Autodesk Fusion 360 part; units mm, degrees
note: some values were not read from the file. Set by a fixed rule: which sketch regions a step uses.
(part 2 of 4)
  line L656 (1.808, 3.3438) -> (1.8184, 3.3438)
  line L657 (1.8184, 3.3438) -> (1.8184, 3.2708)
  line L658 (1.8184, 3.2708) -> (1.9955, 3.2708)
  line L659 (1.1056, 1.5849) -> (1.0838, 1.7478)
  line L660 (0.3556, 1.8201) -> (0.3556, 1.8066)
  line L661 (1.864, 1.1309) -> (1.8639, 1.1244)
  line L662 (3.464, 1.252) -> (3.4045, 1.1285)
  line L663 (3.7483, 1.1867) -> (3.8294, 1.172)
  line L664 (3.8294, 1.172) -> (3.8536, 1.161)
  line L665 (2.3791, 0.7459) -> (2.2162, 0.724)
  line L666 (0.366, 1.8261) -> (0.3556, 1.8261)
  line L667 (1.8639, 1.1244) -> (1.871, 1.0602)
  line L668 (1.871, 1.0602) -> (1.8726, 1.0539)
  line L669 (1.8726, 1.0539) -> (1.874, 1.048)
  line L670 (1.874, 1.048) -> (1.8953, 0.9908)
  line L671 (1.0838, 1.7478) -> (1.0838, 1.8021)
  line L672 (2.3329, 1.4557) -> (2.3298, 1.4598)
  line L673 (2.3298, 1.4599) -> (2.3015, 1.5026)
  line L674 (2.3015, 1.5026) -> (2.2989, 1.507)
  line L675 (3.2523, 0.9032) -> (3.1611, 0.8028)
  line L676 (0.4964, 1.1729) -> (0.5775, 1.1875)
  line L677 (3.24, 1.8201) -> (3.24, 1.8066)
  line L678 (3.5115, 1.3818) -> (3.464, 1.252)
  line L679 (2.2728, 1.5597) -> (2.2674, 1.5779)
  line L680 (2.2674, 1.5779) -> (2.2653, 1.5889)
  line L681 (2.2653, 1.5889) -> (2.2649, 1.5925)
  line L682 (0.9444, 1.8021) -> (0.9444, 1.7407)
  line L683 (3.24, 1.8066) -> (3.24, 1.8021)
  line L684 (3.5463, 1.5173) -> (3.5115, 1.3818)
  line L685 (3.4045, 1.1285) -> (3.3337, 1.0119)
  line L686 (0.3927, 1.8261) -> (0.386, 1.8261)
  line L687 (1.8745, 1.2061) -> (1.8726, 1.1993)
  line L688 (1.8726, 1.1993) -> (1.8712, 1.1937)
  line L689 (1.8712, 1.1937) -> (1.864, 1.1466)
  line L690 (1.864, 1.1466) -> (1.864, 1.1309)
  line L691 (0.7773, 1.5173) -> (0.7559, 1.6576)
  line L692 (1.0838, 1.8216) -> (1.0838, 1.8261)
  line L693 (0.386, 1.8261) -> (0.371, 1.8261)
  line L694 (0.3556, 1.8021) -> (0.3556, 1.7962)
  line L695 (2.4564, 0.0189) -> (2.4958, 0.0258)
  line L696 (2.4958, 0.0258) -> (2.4998, 0.0265)
  line L697 (2.4998, 0.0265) -> (2.4932, 0.0523)
  line L698 (2.4932, 0.0523) -> (2.4928, 0.1347)
  line L699 (0.7559, 1.6576) -> (0.7486, 1.766)
  line L700 (0.6816, 1.1738) -> (0.7743, 1.1242)
  line L701 (0.8122, 1.3818) -> (0.7773, 1.5173)
  line L702 (0.366, 1.8261) -> (0.3556, 1.8261)
  line L703 (3.5751, 1.8261) -> (3.5751, 1.8201)
  line L704 (3.965, 1.8253) -> (3.9235, 1.8257)
  line L705 (3.464, 1.252) -> (3.4045, 1.1285)
  line L706 (2.2611, 3.0885) -> (2.2611, 2.5781)
  line L707 (0.3556, 1.783) -> (0.3556, 1.7787)
  line L708 (1.9446, 0.7459) -> (1.7422, 0.8087)
  line L709 (2.2719, 1.9296) -> (2.0711, 1.9296)
  line L710 (2.0711, 1.9296) -> (2.0684, 1.6354)
  line L711 (2.0684, 1.6354) -> (2.0687, 1.6326)
  line L712 (0.7773, 1.5173) -> (0.7559, 1.6576)
  line L713 (1.3995, 1.0398) -> (1.2679, 1.1993)
  line L714 (2.1075, 0.724) -> (1.9446, 0.7459)
  line L715 (2.3064, 0.3962) -> (2.198, 0.3888)
  line L716 (0.3556, 1.7962) -> (0.3556, 1.783)
  line L717 (0.371, 1.8261) -> (0.366, 1.8261)
  line L718 (2.4467, 0.4176) -> (2.3064, 0.3962)
  line L719 (2.2266, 3.7895) -> (2.2068, 3.8142)
  line L720 (2.2068, 3.8142) -> (2.1871, 3.7895)
  line L721 (2.1871, 3.7895) -> (2.1742, 3.8191)
  line L722 (2.198, 0.3888) -> (2.1619, 0.3888)
  line L723 (0.4557, 1.2069) -> (0.457, 1.2031)
  line L724 (1.8953, 0.9908) -> (1.8981, 0.9854)
  line L725 (1.8981, 0.9854) -> (1.9035, 0.975)
  line L726 (0.7486, 1.8216) -> (0.7486, 1.8261)
  line L727 (2.4467, 0.4176) -> (2.3064, 0.3962)
  line L728 (3.4045, 1.1285) -> (3.3337, 1.0119)
  line L729 (2.3252, 3.8542) -> (2.2951, 3.8553)
  line L730 (2.2951, 3.8553) -> (2.2982, 3.8228)
  line L731 (2.2982, 3.8228) -> (2.2696, 3.8332)
  line L732 (0.9444, 1.8066) -> (0.9444, 1.8021)
  line L733 (2.7647, 0.9081) -> (2.5815, 0.8087)
  line L734 (3.3337, 1.0119) -> (3.2523, 0.9032)
  line L735 (2.2896, 2.7044) -> (2.29, 2.7214)
  line L736 (3.944, 1.7798) -> (3.9705, 1.7778)
  line L737 (3.9705, 1.7778) -> (3.9705, 1.784)
  line L738 (3.9705, 1.784) -> (3.9705, 1.7978)
  line L739 (0.3556, 1.8066) -> (0.3556, 1.8021)
  line L740 (0.8583, 1.019) -> (0.8809, 0.9398)
  line L741 (3.5751, 1.8066) -> (3.5751, 1.8021)
  line L742 (3.5751, 1.8201) -> (3.5751, 1.8066)
  line L743 (3.24, 1.8261) -> (3.24, 1.8201)
  line L744 (1.2679, 1.1993) -> (1.1685, 1.3824)
  line L745 (2.5684, 3.2708) -> (2.5684, 3.3438)
  line L746 (2.5684, 3.3438) -> (2.5788, 3.3438)
  line L747 (2.5788, 3.3438) -> (2.5788, 3.2708)
  line L748 (1.1685, 1.3824) -> (1.1056, 1.5849)
  line L749 (3.5751, 1.8066) -> (3.5751, 1.8021)
  line L750 (2.0174, 0.3962) -> (1.8771, 0.4176)
  line L751 (1.3717, 0.6302) -> (1.2629, 0.7116)
  line L752 (1.7422, 0.8087) -> (1.5591, 0.9081)
  line L753 (2.2649, 1.5925) -> (2.2645, 1.5954)
  line L754 (2.2645, 1.5954) -> (2.2645, 1.624)
  line L755 (2.2645, 1.624) -> (2.2649, 1.6268)
  line L756 (2.1619, 0.724) -> (2.1075, 0.724)
  line L757 (1.1523, 1.1212) -> (1.3011, 0.9409)
  line L758 (2.198, 0.3888) -> (2.1619, 0.3888)
  line L759 (3.6571, 1.5112) -> (3.6617, 1.5374)
  line L760 (3.6617, 1.5374) -> (3.6663, 1.5636)
  line L761 (3.6663, 1.5636) -> (3.6999, 1.6388)
  line L762 (3.6999, 1.6388) -> (3.7698, 1.7171)
  line L763 (0.9691, 1.5566) -> (1.04, 1.3281)
  line L764 (2.0622, 3.9341) -> (2.0863, 3.9538)
  line L765 (2.0863, 3.9538) -> (2.0649, 3.9768)
  line L766 (2.4553, 1.2652) -> (2.4344, 1.308)
  line L767 (1.6881, 0.6799) -> (1.9167, 0.6089)
  line L768 (2.0995, 3.8845) -> (2.0702, 3.8922)
  line L769 (2.0702, 3.8922) -> (2.0885, 3.9181)
  line L770 (2.0885, 3.9181) -> (2.0622, 3.9341)
  line L771 (3.0608, 0.7116) -> (2.952, 0.6302)
  line L772 (2.0762, 2.5171) -> (2.2852, 2.5171)
  line L773 (2.0945, 2.5781) -> (2.0945, 3.0885)
  line L774 (2.2611, 2.5781) -> (2.0945, 2.5781)
  line L775 (2.2142, 2.8333) -> (2.0892, 2.8333)
  line L776 (0.99, 1.0119) -> (0.9192, 1.1285)
  line L777 (2.712, 0.4999) -> (2.5821, 0.4524)
  line L778 (3.9705, 1.8081) -> (3.9692, 1.8236)
  line L779 (3.9692, 1.8236) -> (3.9692, 1.8255)
  line L780 (2.2611, 2.5781) -> (2.0945, 2.5781)
  line L781 (0.9192, 1.1285) -> (0.8596, 1.252)
  line L782 (3.1611, 0.8028) -> (3.0608, 0.7116)
  line L783 (1.4813, 0.7922) -> (1.6881, 0.6799)
  line L784 (2.1153, 3.8228) -> (2.1185, 3.8553)
  line L785 (2.1185, 3.8553) -> (2.0883, 3.8542)
  line L786 (2.0883, 3.8542) -> (2.0995, 3.8845)
  line L787 (0.6691, 1.5119) -> (0.6631, 1.4297)
  line L788 (3.773, 1.2543) -> (3.7021, 1.3317)
  line L789 (3.7021, 1.3317) -> (3.663, 1.4291)
  line L790 (3.663, 1.4291) -> (3.6571, 1.5112)
  line L791 (1.2629, 0.7116) -> (1.1625, 0.8028)
  line L792 (0.9444, 1.7407) -> (0.9691, 1.5566)
  line L793 (2.1641, 3.1785) -> (2.1812, 3.1785)
  line L794 (2.9242, 1.0398) -> (2.7647, 0.9081)
  line L795 (3.8536, 1.161) -> (3.855, 1.1648)
  line L796 (3.855, 1.1648) -> (3.8688, 1.2024)
  line L797 (3.8688, 1.2024) -> (3.8701, 1.2062)
  line L798 (1.6118, 0.4999) -> (1.4882, 0.5595)
  line L799 (2.1619, 0.3888) -> (2.1258, 0.3888)
  line L800 (2.1742, 3.8191) -> (2.1491, 3.8011)
  line L801 (2.1491, 3.8011) -> (2.144, 3.8332)
  line L802 (2.144, 3.8332) -> (2.1153, 3.8228)
  line L803 (2.8355, 0.5595) -> (2.712, 0.4999)
  line L804 (2.952, 0.6302) -> (2.8355, 0.5595)
  line L805 (2.0038, 1.0902) -> (2.0042, 1.1043)
  line L806 (2.0042, 1.1043) -> (2.0103, 1.1212)
  line L807 (2.0103, 1.1212) -> (2.0221, 1.1346)
  line L808 (2.0221, 1.1346) -> (2.0342, 1.1418)
  line L809 (2.1008, 0.5841) -> (2.1622, 0.584)
  line L810 (2.5821, 0.4524) -> (2.4467, 0.4176)
  line L811 (2.2852, 2.5171) -> (2.2856, 2.5341)
  line L812 (2.0342, 1.1418) -> (2.0386, 1.143)
  line L813 (2.7402, 3.4792) -> (1.6257, 3.4792)
  line L814 (2.0174, 0.3962) -> (1.8771, 0.4176)
  line L815 (2.0386, 1.143) -> (2.2912, 1.2032)
  line L816 (2.2912, 1.2032) -> (2.2956, 1.2042)
  line L817 (2.2956, 1.2042) -> (2.3094, 1.2032)
  line L818 (2.3094, 1.2032) -> (2.3255, 1.1962)
  line L819 (1.7416, 0.4524) -> (1.6118, 0.4999)
  line L820 (3.3337, 1.0119) -> (3.2523, 0.9032)
  line L821 (2.1614, 2.4099) -> (2.1679, 2.4043)
  line L822 (2.1903, 2.2499) -> (2.171, 2.2289)
  line L823 (3.8294, 1.172) -> (3.8536, 1.161)
  line L824 (2.1622, 0.584) -> (2.2235, 0.584)
  line L825 (3.4449, 0.9392) -> (3.4676, 1.0185)
  line L826 (2.4219, 0.1221) -> (2.4498, 0.0447)
  line L827 (3.6617, 1.5374) -> (3.6663, 1.5636)
  line L828 (3.2844, 1.328) -> (3.3554, 1.5566)
  line L829 (3.7021, 1.3317) -> (3.663, 1.4291)
  line L830 (3.1722, 1.1211) -> (3.2844, 1.328)
  line L831 (3.3554, 1.5566) -> (3.3802, 1.7407)
  line L832 (1.9287, 1.3096) -> (1.9117, 1.2848)
  line L833 (1.9117, 1.2848) -> (1.9067, 1.2763)
  line L834 (1.9067, 1.2763) -> (1.9029, 1.2703)
  line L835 (1.9029, 1.2703) -> (1.8745, 1.2061)
  line L836 (2.4076, 0.6088) -> (2.6363, 0.6798)
  line L837 (3.663, 1.4291) -> (3.6571, 1.5112)
  line L838 (2.1208, 2.4293) -> (2.1614, 2.4099)
  line L839 (2.0737, 2.4375) -> (2.1208, 2.4293)
  line L840 (3.3802, 1.8081) -> (3.3802, 1.8216)
  line L841 (3.3802, 1.8216) -> (3.3802, 1.8261)
  line L842 (2.0279, 2.3502) -> (1.97, 2.3502)
  line L843 (3.9915, 2.0278) -> (3.9915, 2.4375)
  line L844 (2.0728, 2.2944) -> (2.0763, 2.3079)
  line L845 (2.0642, 2.2834) -> (2.0728, 2.2944)
  line L846 (1.97, 2.3502) -> (1.97, 2.2719)
  line L847 (3.4656, 2.2733) -> (3.4656, 2.1809)
  line L848 (4.1268, 2.2083) -> (4.1227, 2.2152)
  line L849 (4.1101, 2.4375) -> (4.2055, 2.2875)
  line L850 (3.3321, 2.34) -> (3.3321, 2.2733)
  line L851 (3.3321, 2.2733) -> (3.4656, 2.2733)
  line L852 (4.2457, 2.2157) -> (4.2488, 2.2089)
  line L853 (2.0763, 2.3079) -> (2.0762, 2.3108)
  line L854 (4.2389, 2.0276) -> (4.1268, 2.2083)
  line L855 (3.8622, 2.1926) -> (3.7128, 2.1926)
  line L856 (2.4376, 2.4375) -> (2.4376, 2.2869)
  line L857 (4.2096, 2.2812) -> (4.2457, 2.2157)
  line L858 (4.2488, 2.2089) -> (4.2471, 2.2178)
  line L859 (2.9999, 2.4375) -> (3.1283, 2.0279)
  line L860 (3.8976, 2.0272) -> (3.5892, 2.0272)
  line L861 (2.027, 2.2717) -> (2.0589, 2.28)
  line L862 (2.9217, 2.3168) -> (2.8886, 2.1979)
  line L863 (4.3412, 2.0276) -> (4.2389, 2.0276)
  line L864 (3.3321, 2.0276) -> (3.2097, 2.0276)
  line L865 (3.8976, 2.4375) -> (3.8976, 2.343)
  line L866 (2.8669, 2.4375) -> (2.9999, 2.4375)
  line L867 (2.0641, 2.3404) -> (2.0369, 2.3502)
  line L868 (2.0762, 2.3108) -> (2.0762, 2.3182)
  line L869 (2.1345, 2.2065) -> (2.2089, 2.0276)
  line L870 (2.5336, 2.1869) -> (2.4376, 2.1869)
  line L871 (4.2392, 2.3163) -> (4.2392, 2.4375)
  line L872 (4.2392, 2.4375) -> (4.3415, 2.4375)
  line L873 (4.2055, 2.2875) -> (4.2096, 2.2812)
  line L874 (2.1418, 2.21) -> (2.1345, 2.2065)
  line L875 (4.2392, 2.2917) -> (4.2392, 2.3163)
  line L876 (4.2471, 2.2178) -> (4.2392, 2.2917)
  line L877 (4.0936, 2.0278) -> (3.9915, 2.0278)
  line L878 (2.0369, 2.3502) -> (2.0279, 2.3502)
  line L879 (3.1283, 2.0279) -> (3, 2.0276)
  line L880 (4.3415, 2.4375) -> (4.3412, 2.0276)
  line L881 (2.0762, 2.3182) -> (2.0641, 2.3404)
  line L882 (2.171, 2.2289) -> (2.1418, 2.21)
  line L883 (2.0618, 2.2818) -> (2.0642, 2.2834)
  line L884 (2.0589, 2.28) -> (2.0618, 2.2818)
  line L885 (3.9915, 2.4375) -> (4.1101, 2.4375)
  line L886 (2.0558, 0.2607) -> (2.1356, 0.2808)
  line L887 (2.1889, 0.2808) -> (2.2687, 0.2607)
  line L888 (3.6663, 1.5636) -> (3.6999, 1.6388)
  line L889 (3.8688, 1.2024) -> (3.8701, 1.2062)
  line L890 (3.6999, 1.6388) -> (3.7698, 1.7171)
  line L891 (2.1744, 2.399) -> (2.1976, 2.3652)
  line L892 (2.1976, 2.3652) -> (2.2074, 2.3253)
  line L893 (2.1679, 2.4043) -> (2.1744, 2.399)
  line L894 (2.9548, 2.1979) -> (2.9217, 2.3168)
  line L895 (3.7128, 2.1926) -> (3.7128, 2.125)
  line L896 (4.0847, 2.2874) -> (4.0934, 2.2314)
  line L897 (3.5892, 2.0272) -> (3.5892, 2.4375)
  line L898 (3.5892, 2.4375) -> (3.8976, 2.4375)
  line L899 (2.3119, 2.0276) -> (2.3119, 2.4375)
  line L900 (3.8976, 2.343) -> (3.7128, 2.343)
  line L901 (3.2097, 2.4375) -> (3.5059, 2.4375)
  line L902 (4.1227, 2.2152) -> (4.0864, 2.2856)
  line L903 (4.0864, 2.2856) -> (4.0832, 2.2929)
  line L904 (2.5336, 2.2869) -> (2.5336, 2.4375)
  line L905 (3.7128, 2.2835) -> (3.8622, 2.2835)
  line L906 (4.0832, 2.2929) -> (4.0847, 2.2874)
  line L907 (2.4376, 2.0276) -> (2.3119, 2.0276)
  line L908 (2.4376, 2.2869) -> (2.5336, 2.2869)
  line L909 (2.3119, 2.4375) -> (2.4376, 2.4375)
  line L910 (4.0934, 2.2314) -> (4.0936, 2.2258)
  line L911 (2.4376, 2.1869) -> (2.4376, 2.0276)
  line L912 (2.5336, 2.0279) -> (2.5336, 2.1868)
  line L913 (2.6594, 2.0279) -> (2.5336, 2.0279)
  line L914 (2.7404, 2.0276) -> (2.8669, 2.4375)
  line L915 (3.7128, 2.125) -> (3.8976, 2.125)
  line L916 (2.8671, 2.1084) -> (2.8425, 2.0276)
  line L917 (3.8622, 2.2835) -> (3.8622, 2.1926)
  line L918 (2.8425, 2.0276) -> (2.7404, 2.0276)
  line L919 (3.0234, 0.9408) -> (3.1722, 1.1211)
  line L920 (3.9705, 1.8023) -> (3.9705, 1.8081)
  line L921 (2.2235, 0.584) -> (2.4076, 0.6088)
  line L922 (3.0453, 0.2249) -> (3.0488, 0.2268)
  line L923 (3.9692, 1.8236) -> (3.9692, 1.8255)
  line L924 (2.8432, 0.7921) -> (3.0234, 0.9408)
  line L925 (3.5059, 2.4375) -> (3.5059, 2.34)
  line L926 (3.5059, 2.34) -> (3.3321, 2.34)
  line L927 (2.6363, 0.6798) -> (2.8432, 0.7921)
  line L928 (3.9705, 1.784) -> (3.9705, 1.7978)
sketch "Sketch8" plane through (0, 0, 0) normal (0, 1, 0) x (1, 0, 0)
  line L0 (73.512, 49.4274) -> (73.512, 49.3184)
  line L1 (73.512, 49.3184) -> (73.4165, 49.3254)
  line L2 (73.4165, 49.3254) -> (73.1245, 49.2746)
  line L3 (73.1245, 49.2746) -> (72.7894, 49.0999)
  line L4 (72.7894, 49.0999) -> (72.5376, 48.8178)
  line L5 (72.5376, 48.8178) -> (72.4167, 48.5471)
  line L6 (72.4167, 48.5471) -> (72.4004, 48.4528)
  line L7 (72.4004, 48.4528) -> (72.3837, 48.3587)
  line L8 (72.3837, 48.3587) -> (72.405, 48.0631)
  line L9 (72.405, 48.0631) -> (72.5457, 47.7121)
  line L10 (72.5457, 47.7121) -> (72.8009, 47.4336)
  line L11 (72.8009, 47.4336) -> (73.0582, 47.2864)
  line L12 (73.0582, 47.2864) -> (73.1505, 47.2604)
  line L13 (73.1505, 47.2604) -> (73.1456, 47.2469)
  line L14 (73.1456, 47.2469) -> (73.0962, 47.1115)
  line L15 (73.0962, 47.1115) -> (73.0912, 47.0979)
  line L16 (73.0912, 47.0979) -> (73.0038, 47.1375)
  line L17 (73.0038, 47.1375) -> (72.7121, 47.1903)
  line L18 (72.7121, 47.1903) -> (72.3373, 47.1414)
  line L19 (72.3373, 47.1414) -> (72.0039, 46.9631)
  line L20 (72.0039, 46.9631) -> (71.7972, 46.7504)
  line L21 (71.7972, 46.7504) -> (71.7493, 46.6674)
  line L22 (71.7493, 46.6674) -> (71.7013, 46.5846)
  line L23 (71.7013, 46.5846) -> (71.6199, 46.2994)
  line L24 (71.6199, 46.2994) -> (71.6314, 45.9215)
  line L25 (71.6314, 45.9215) -> (71.7757, 45.5721)
  line L26 (71.7757, 45.5721) -> (71.9667, 45.3453)
  line L27 (71.9667, 45.3453) -> (72.0447, 45.2893)
  line L28 (72.0447, 45.2893) -> (72.0353, 45.2782)
  line L29 (72.0353, 45.2782) -> (71.9415, 45.1682)
  line L30 (71.9415, 45.1682) -> (71.9322, 45.1573)
  line L31 (71.9322, 45.1573) -> (71.8634, 45.2244)
  line L32 (71.8634, 45.2244) -> (71.6071, 45.3737)
  line L33 (71.6071, 45.3737) -> (71.238, 45.4557)
  line L34 (71.238, 45.4557) -> (70.8636, 45.402)
  line L35 (70.8636, 45.402) -> (70.5968, 45.2725)
  line L36 (70.5968, 45.2725) -> (70.5234, 45.2108)
  line L37 (70.5234, 45.2108) -> (70.45, 45.1493)
  line L38 (70.45, 45.1493) -> (70.2759, 44.9088)
  line L39 (70.2759, 44.9088) -> (70.158, 44.5494)
  line L40 (70.158, 44.5494) -> (70.1746, 44.1717)
  line L41 (70.1746, 44.1717) -> (70.2771, 43.8934)
  line L42 (70.2771, 43.8934) -> (70.3312, 43.8141)
  line L43 (70.3312, 43.8141) -> (70.3185, 43.8067)
  line L44 (70.3185, 43.8067) -> (70.1937, 43.7348)
  line L45 (70.1937, 43.7348) -> (70.1812, 43.7278)
  line L46 (70.1812, 43.7278) -> (70.1396, 43.8143)
  line L47 (70.1396, 43.8143) -> (69.95, 44.0422)
  line L48 (69.95, 44.0422) -> (69.631, 44.2457)
  line L49 (69.631, 44.2457) -> (69.2607, 44.3233)
  line L50 (69.2607, 44.3233) -> (68.9658, 44.293)
  line L51 (68.9658, 44.293) -> (68.8757, 44.2602)
  line L52 (68.8757, 44.2602) -> (68.7855, 44.2276)
  line L53 (68.7855, 44.2276) -> (68.54, 44.0612)
  line L54 (68.54, 44.0612) -> (68.3062, 43.7637)
  line L55 (68.3062, 43.7637) -> (68.1923, 43.403)
  line L56 (68.1923, 43.403) -> (68.1935, 43.1065)
  line L57 (68.1935, 43.1065) -> (68.2173, 43.0135)
  line L58 (68.2173, 43.0135) -> (68.2028, 43.011)
  line L59 (68.2028, 43.011) -> (68.0613, 42.9862)
  line L60 (68.0613, 42.9862) -> (68.047, 42.9838)
  line L61 (68.047, 42.9838) -> (68.0375, 43.0791)
  line L62 (68.0375, 43.0791) -> (67.9369, 43.3578)
  line L63 (67.9369, 43.3578) -> (67.7068, 43.6576)
  line L64 (67.7068, 43.6576) -> (67.3855, 43.8569)
  line L65 (67.3855, 43.8569) -> (67.098, 43.9289)
  line L66 (67.098, 43.9289) -> (66.9064, 43.9289)
  line L67 (66.9064, 43.9289) -> (66.6191, 43.8569)
  line L68 (66.6191, 43.8569) -> (66.2978, 43.6576)
  line L69 (66.2978, 43.6576) -> (66.0675, 43.3578)
  line L70 (66.0675, 43.3578) -> (65.9671, 43.0791)
  line L71 (65.9671, 43.0791) -> (65.9576, 42.9838)
  line L72 (65.9576, 42.9838) -> (65.9431, 42.9862)
  line L73 (65.9431, 42.9862) -> (65.8017, 43.011)
  line L74 (65.8017, 43.011) -> (65.7877, 43.0135)
  line L75 (65.7877, 43.0135) -> (65.8115, 43.1065)
  line L76 (65.8115, 43.1065) -> (65.8127, 43.403)
  line L77 (65.8127, 43.403) -> (65.6994, 43.7639)
  line L78 (65.6994, 43.7639) -> (65.4655, 44.0614)
  line L79 (65.4655, 44.0614) -> (65.2201, 44.228)
  line L80 (65.2201, 44.228) -> (65.13, 44.2606)
  line L81 (65.13, 44.2606) -> (65.0398, 44.2934)
  line L82 (65.0398, 44.2934) -> (64.7449, 44.3241)
  line L83 (64.7449, 44.3241) -> (64.3746, 44.2467)
  line L84 (64.3746, 44.2467) -> (64.0554, 44.0434)
  line L85 (64.0554, 44.0434) -> (63.8656, 43.8155)
  line L86 (63.8656, 43.8155) -> (63.8242, 43.7289)
  line L87 (63.8242, 43.7289) -> (63.8113, 43.736)
  line L88 (63.8113, 43.736) -> (63.6865, 43.8078)
  line L89 (63.6865, 43.8078) -> (63.6741, 43.8153)
  line L90 (63.6741, 43.8153) -> (63.7281, 43.8944)
  line L91 (63.7281, 43.8944) -> (63.8306, 44.1727)
  line L92 (63.8306, 44.1727) -> (63.8474, 44.5504)
  line L93 (63.8474, 44.5504) -> (63.7296, 44.9098)
  line L94 (63.7296, 44.9098) -> (63.5558, 45.15)
  line L95 (63.5558, 45.15) -> (63.4826, 45.2116)
  line L96 (63.4826, 45.2116) -> (63.4091, 45.2733)
  line L97 (63.4091, 45.2733) -> (63.1425, 45.403)
  line L98 (63.1425, 45.403) -> (62.7683, 45.4569)
  line L99 (62.7683, 45.4569) -> (62.399, 45.3752)
  line L100 (62.399, 45.3752) -> (62.1427, 45.2262)
  line L101 (62.1427, 45.2262) -> (62.0742, 45.1592)
  line L102 (62.0742, 45.1592) -> (62.0648, 45.1701)
  line L103 (62.0648, 45.1701) -> (61.9724, 45.2805)
  line L104 (61.9724, 45.2805) -> (61.9634, 45.2916)
  line L105 (61.9634, 45.2916) -> (62.0411, 45.3477)
  line L106 (62.0411, 45.3477) -> (62.2326, 45.5742)
  line L107 (62.2326, 45.5742) -> (62.3773, 45.9235)
  line L108 (62.3773, 45.9235) -> (62.3892, 46.3016)
  line L109 (62.3892, 46.3016) -> (62.3079, 46.5867)
  line L110 (62.3079, 46.5867) -> (62.2601, 46.6696)
  line L111 (62.2601, 46.6696) -> (62.212, 46.7526)
  line L112 (62.212, 46.7526) -> (62.0054, 46.9655)
  line L113 (62.0054, 46.9655) -> (61.672, 47.144)
  line L114 (61.672, 47.144) -> (61.297, 47.1932)
  line L115 (61.297, 47.1932) -> (61.0052, 47.1407)
  line L116 (61.0052, 47.1407) -> (60.9179, 47.101)
  line L117 (60.9179, 47.101) -> (60.9124, 47.1145)
  line L118 (60.9124, 47.1145) -> (60.8634, 47.2495)
  line L119 (60.8634, 47.2495) -> (60.8587, 47.2629)
  line L120 (60.8587, 47.2629) -> (60.9509, 47.2887)
  line L121 (60.9509, 47.2887) -> (61.2083, 47.4358)
  line L122 (61.2083, 47.4358) -> (61.4642, 47.7143)
  line L123 (61.4642, 47.7143) -> (61.6052, 48.0653)
  line L124 (61.6052, 48.0653) -> (61.6269, 48.361)
  line L125 (61.6269, 48.361) -> (61.6105, 48.4553)
  line L126 (61.6105, 48.4553) -> (61.5939, 48.5499)
  line L127 (61.5939, 48.5499) -> (61.473, 48.8205)
  line L128 (61.473, 48.8205) -> (61.2212, 49.1027)
  line L129 (61.2212, 49.1027) -> (60.8859, 49.2777)
  line L130 (60.8859, 49.2777) -> (60.5939, 49.3285)
  line L131 (60.5939, 49.3285) -> (60.4984, 49.3213)
  line L132 (60.4984, 49.3213) -> (60.4984, 49.492)
  line L133 (60.4984, 49.492) -> (61.9132, 49.492)
  line L134 (61.9132, 49.492) -> (61.9132, 49.2758)
  line L135 (61.9132, 49.2758) -> (61.9394, 48.8856)
  line L136 (61.9394, 48.8856) -> (62.0165, 48.3805)
  line L137 (62.0165, 48.3805) -> (62.1419, 47.8928)
  line L138 (62.1419, 47.8928) -> (62.3128, 47.4254)
  line L139 (62.3128, 47.4254) -> (62.5271, 46.9807)
  line L140 (62.5271, 46.9807) -> (62.782, 46.5612)
  line L141 (62.782, 46.5612) -> (63.0749, 46.1696)
  line L142 (63.0749, 46.1696) -> (63.4032, 45.8082)
  line L143 (63.4032, 45.8082) -> (63.7646, 45.4799)
  line L144 (63.7646, 45.4799) -> (64.1562, 45.1869)
  line L145 (64.1562, 45.1869) -> (64.5757, 44.9323)
  line L146 (64.5757, 44.9323) -> (65.0204, 44.718)
  line L147 (65.0204, 44.718) -> (65.4879, 44.5469)
  line L148 (65.4879, 44.5469) -> (65.9755, 44.4215)
  line L149 (65.9755, 44.4215) -> (66.4806, 44.3444)
  line L150 (66.4806, 44.3444) -> (66.8708, 44.318)
  line L151 (66.8708, 44.318) -> (67.1308, 44.318)
  line L152 (67.1308, 44.318) -> (67.5211, 44.3444)
  line L153 (67.5211, 44.3444) -> (68.0261, 44.4215)
  line L154 (68.0261, 44.4215) -> (68.5136, 44.5469)
  line L155 (68.5136, 44.5469) -> (68.9812, 44.718)
  line L156 (68.9812, 44.718) -> (69.4259, 44.9323)
  line L157 (69.4259, 44.9323) -> (69.8453, 45.1869)
  line L158 (69.8453, 45.1869) -> (70.2368, 45.4799)
  line L159 (70.2368, 45.4799) -> (70.5982, 45.8082)
  line L160 (70.5982, 45.8082) -> (70.9265, 46.1696)
  line L161 (70.9265, 46.1696) -> (71.2195, 46.5612)
  line L162 (71.2195, 46.5612) -> (71.4743, 46.9807)
  line L163 (71.4743, 46.9807) -> (71.6886, 47.4254)
  line L164 (71.6886, 47.4254) -> (71.8595, 47.8928)
  line L165 (71.8595, 47.8928) -> (71.9849, 48.3805)
  line L166 (71.9849, 48.3805) -> (72.062, 48.8856)
  line L167 (72.062, 48.8856) -> (72.0884, 49.2758)
  line L168 (72.0884, 49.2758) -> (72.0884, 49.492)
  line L169 (72.0884, 49.492) -> (73.3279, 49.492)
  line L170 (73.3279, 49.492) -> (73.3427, 49.4906)
  line L171 (73.3427, 49.4906) -> (73.4921, 49.4891)
  line L172 (73.4921, 49.4891) -> (73.5072, 49.4901)
  line L173 (73.5072, 49.4901) -> (73.5072, 49.483)
  line L174 (73.5072, 49.483) -> (73.512, 49.4274)
  line L175 (69.4534, 45.7698) -> (68.7087, 45.3655)
  line L176 (68.7087, 45.3655) -> (67.8855, 45.11)
  line L177 (67.8855, 45.11) -> (67.2228, 45.0207)
  line L178 (67.2228, 45.0207) -> (67.0019, 45.0207)
  line L179 (67.0019, 45.0207) -> (66.781, 45.0209)
  line L180 (66.781, 45.0209) -> (66.1183, 45.1102)
  line L181 (66.1183, 45.1102) -> (65.2953, 45.3657)
  line L182 (65.2953, 45.3657) -> (64.5507, 45.77)
  line L183 (64.5507, 45.77) -> (63.9019, 46.3055)
  line L184 (63.9019, 46.3055) -> (63.3665, 46.9543)
  line L185 (63.3665, 46.9543) -> (62.9622, 47.6992)
  line L186 (62.9622, 47.6992) -> (62.707, 48.5221)
  line L187 (62.707, 48.5221) -> (62.6179, 49.1848)
  line L188 (62.6179, 49.1848) -> (62.6179, 49.492)
  line L189 (62.6179, 49.492) -> (63.1197, 49.492)
  line L190 (63.1197, 49.492) -> (63.1197, 49.2102)
  line L191 (63.1197, 49.2102) -> (63.1984, 48.6237)
  line L192 (63.1984, 48.6237) -> (63.4246, 47.8949)
  line L193 (63.4246, 47.8949) -> (63.7824, 47.2358)
  line L194 (63.7824, 47.2358) -> (64.2564, 46.6614)
  line L195 (64.2564, 46.6614) -> (64.8308, 46.1873)
  line L196 (64.8308, 46.1873) -> (65.49, 45.8295)
  line L197 (65.49, 45.8295) -> (66.2187, 45.6033)
  line L198 (66.2187, 45.6033) -> (66.8052, 45.5244)
  line L199 (66.8052, 45.5244) -> (67.1964, 45.5244)
  line L200 (67.1964, 45.5244) -> (67.7829, 45.6033)
  line L201 (67.7829, 45.6033) -> (68.5116, 45.8295)
  line L202 (68.5116, 45.8295) -> (69.1708, 46.1873)
  line L203 (69.1708, 46.1873) -> (69.7453, 46.6614)
  line L204 (69.7453, 46.6614) -> (70.2192, 47.2358)
  line L205 (70.2192, 47.2358) -> (70.5771, 47.8949)
  line L206 (70.5771, 47.8949) -> (70.8033, 48.6237)
  line L207 (70.8033, 48.6237) -> (70.8821, 49.2102)
  line L208 (70.8821, 49.2102) -> (70.8821, 49.492)
  line L209 (70.8821, 49.492) -> (71.3869, 49.492)
  line L210 (71.3869, 49.492) -> (71.3869, 49.1848)
  line L211 (71.3869, 49.1848) -> (71.2976, 48.5221)
  line L212 (71.2976, 48.5221) -> (71.0421, 47.6991)
  line L213 (71.0421, 47.6991) -> (70.6378, 46.9541)
  line L214 (70.6378, 46.9541) -> (70.1025, 46.3051)
  line L215 (70.1025, 46.3051) -> (69.4534, 45.7698)
  line L216 (65.9662, 47.2602) -> (66.0685, 47.4914)
  line L217 (66.0685, 47.4914) -> (66.0822, 47.5127)
  line L218 (66.0822, 47.5127) -> (66.1004, 47.5436)
  line L219 (66.1004, 47.5436) -> (66.1615, 47.6326)
  line L220 (66.1615, 47.6326) -> (66.224, 47.7063)
  line L221 (66.224, 47.7063) -> (66.2845, 47.7756)
  line L222 (66.2845, 47.7756) -> (66.341, 47.8545)
  line L223 (66.341, 47.8545) -> (66.3578, 47.8821)
  line L224 (66.3578, 47.8821) -> (66.3763, 47.9139)
  line L225 (66.3763, 47.9139) -> (66.5298, 48.2475)
  line L226 (66.5298, 48.2475) -> (66.5419, 48.2822)
  line L227 (66.5419, 48.2822) -> (66.5457, 48.2932)
  line L228 (66.5457, 48.2932) -> (66.5567, 48.326)
  line L229 (66.5567, 48.326) -> (66.567, 48.3584)
  line L230 (66.567, 48.3584) -> (66.5796, 48.3991)
  line L231 (66.5796, 48.3991) -> (66.597, 48.4502)
  line L232 (66.597, 48.4502) -> (66.6031, 48.4671)
  line L233 (66.6031, 48.4671) -> (66.6103, 48.4844)
  line L234 (66.6103, 48.4844) -> (66.6615, 48.6639)
  line L235 (66.6615, 48.6639) -> (66.6644, 48.6822)
  line L236 (66.6644, 48.6822) -> (66.6654, 48.6926)
  line L237 (66.6654, 48.6926) -> (66.6654, 48.7956)
  line L238 (66.6654, 48.7956) -> (66.6644, 48.8057)
  line L239 (66.6644, 48.8057) -> (66.6742, 49.8647)
  line L240 (66.6742, 49.8647) -> (67.3968, 49.8647)
  line L241 (67.3968, 49.8647) -> (67.3946, 49.7739)
  line L242 (67.3946, 49.7739) -> (67.3738, 48.8656)
  line L243 (67.3738, 48.8656) -> (67.3718, 48.7746)
  line L244 (67.3718, 48.7746) -> (67.3704, 48.7645)
  line L245 (67.3704, 48.7645) -> (67.3704, 48.6615)
  line L246 (67.3704, 48.6615) -> (67.3718, 48.6512)
  line L247 (67.3718, 48.6512) -> (67.3732, 48.6381)
  line L248 (67.3732, 48.6381) -> (67.3806, 48.5985)
  line L249 (67.3806, 48.5985) -> (67.4001, 48.533)
  line L250 (67.4001, 48.533) -> (67.4363, 48.4498)
  line L251 (67.4363, 48.4498) -> (67.4788, 48.3695)
  line L252 (67.4788, 48.3695) -> (67.4943, 48.3434)
  line L253 (67.4943, 48.3434) -> (67.5035, 48.3276)
  line L254 (67.5035, 48.3276) -> (67.6054, 48.1737)
  line L255 (67.6054, 48.1737) -> (67.6165, 48.1589)
  line L256 (67.6165, 48.1589) -> (67.6464, 48.1217)
  line L257 (67.6464, 48.1217) -> (67.7341, 48.0078)
  line L258 (67.7341, 48.0078) -> (67.8618, 47.8266)
  line L259 (67.8618, 47.8266) -> (67.9819, 47.627)
  line L260 (67.9819, 47.627) -> (68.0571, 47.4731)
  line L261 (68.0571, 47.4731) -> (68.0767, 47.4197)
  line L262 (68.0767, 47.4197) -> (68.0751, 47.4182)
  line L263 (68.0751, 47.4182) -> (68.097, 47.3567)
  line L264 (68.097, 47.3567) -> (68.1489, 47.0371)
  line L265 (68.1489, 47.0371) -> (68.1241, 46.7147)
  line L266 (68.1241, 46.7147) -> (68.1075, 46.6514)
  line L267 (68.1075, 46.6514) -> (68.0974, 46.6147)
  line L268 (68.0974, 46.6147) -> (68.0593, 46.5061)
  line L269 (68.0593, 46.5061) -> (67.995, 46.361)
  line L270 (67.995, 46.361) -> (67.9214, 46.2403)
  line L271 (67.9214, 46.2403) -> (67.8673, 46.1801)
  line L272 (67.8673, 46.1801) -> (67.8451, 46.1684)
  line L273 (67.8451, 46.1684) -> (67.8451, 46.177)
  line L274 (67.8451, 46.177) -> (67.8418, 46.2028)
  line L275 (67.8418, 46.2028) -> (67.8411, 46.2059)
  line L276 (67.8411, 46.2059) -> (67.6568, 47.1178)
  line L277 (67.6568, 47.1178) -> (67.6543, 47.1336)
  line L278 (67.6543, 47.1336) -> (67.6336, 47.1791)
  line L279 (67.6336, 47.1791) -> (67.5898, 47.2246)
  line L280 (67.5898, 47.2246) -> (67.5319, 47.2496)
  line L281 (67.5319, 47.2496) -> (67.4822, 47.2532)
  line L282 (67.4822, 47.2532) -> (67.4666, 47.2498)
  line L283 (67.4666, 47.2498) -> (66.5572, 47.033)
  line L284 (66.5572, 47.033) -> (66.5414, 47.0285)
  line L285 (66.5414, 47.0285) -> (66.4976, 47.0028)
  line L286 (66.4976, 47.0028) -> (66.4552, 46.9543)
  line L287 (66.4552, 46.9543) -> (66.4334, 46.8936)
  line L288 (66.4334, 46.8936) -> (66.432, 46.8428)
  line L289 (66.432, 46.8428) -> (66.4357, 46.8268)
  line L290 (66.4357, 46.8268) -> (66.6202, 45.9149)
  line L291 (66.6202, 45.9149) -> (66.6205, 45.9141)
  line L292 (66.6205, 45.9141) -> (66.6232, 45.9053)
  line L293 (66.6232, 45.9053) -> (66.6236, 45.9043)
  line L294 (66.6236, 45.9043) -> (66.6142, 45.9094)
  line L295 (66.6142, 45.9094) -> (66.5205, 45.9676)
  line L296 (66.5205, 45.9676) -> (66.5111, 45.9744)
  line L297 (66.5111, 45.9744) -> (66.4946, 45.9862)
  line L298 (66.4946, 45.9862) -> (66.3411, 46.1143)
  line L299 (66.3411, 46.1143) -> (66.3269, 46.1282)
  line L300 (66.3269, 46.1282) -> (66.3011, 46.1528)
  line L301 (66.3011, 46.1528) -> (66.1796, 46.2776)
  line L302 (66.1796, 46.2776) -> (66.0708, 46.4282)
  line L303 (66.0708, 46.4282) -> (66.0513, 46.4657)
  line L304 (66.0513, 46.4657) -> (66.0411, 46.4852)
  line L305 (66.0411, 46.4852) -> (65.9646, 46.6909)
  line L306 (65.9646, 46.6909) -> (65.9595, 46.7121)
  line L307 (65.9595, 46.7121) -> (65.9538, 46.7348)
  line L308 (65.9538, 46.7348) -> (65.9283, 46.966)
  line L309 (65.9283, 46.966) -> (65.9286, 46.9893)
  line L310 (65.9286, 46.9893) -> (65.9286, 47.0459)
  line L311 (65.9286, 47.0459) -> (65.9542, 47.2154)
  line L312 (65.9542, 47.2154) -> (65.9595, 47.2356)
  line L313 (65.9595, 47.2356) -> (65.9662, 47.2602)
  line L314 (67.4463, 52.0411) -> (67.4449, 51.9797)
  line L315 (67.4449, 51.9797) -> (66.6923, 51.9797)
  line L316 (66.6923, 51.9797) -> (66.6939, 52.184)
  line L317 (66.6939, 52.184) -> (66.7113, 54.2264)
  line L318 (66.7113, 54.2264) -> (66.7132, 54.4307)
  line L319 (66.7132, 54.4307) -> (67.4946, 54.4307)
  line L320 (67.4946, 54.4307) -> (67.4621, 52.7151)
  line L321 (67.4621, 52.7151) -> (67.4605, 52.6539)
  line L322 (67.4605, 52.6539) -> (67.4463, 52.0411)
  line L323 (65.0483, 55.4432) -> (69.1046, 55.4432)
  line L324 (69.1046, 55.4432) -> (69.1701, 55.4252)
  line L325 (69.1701, 55.4252) -> (69.2412, 55.377)
  line L326 (69.2412, 55.377) -> (69.2892, 55.3057)
  line L327 (69.2892, 55.3057) -> (69.3067, 55.2401)
  line L328 (69.3067, 55.2401) -> (69.3067, 54.9158)
  line L329 (69.3067, 54.9158) -> (69.3066, 54.8954)
  line L330 (69.3066, 54.8954) -> (69.2905, 54.8338)
  line L331 (69.2905, 54.8338) -> (69.2472, 54.7651)
  line L332 (69.2472, 54.7651) -> (69.1824, 54.7163)
  line L333 (69.1824, 54.7163) -> (69.1222, 54.6952)
  line L334 (69.1222, 54.6952) -> (69.1019, 54.6932)
  line L335 (69.1019, 54.6932) -> (69.1019, 55.2182)
  line L336 (69.1019, 55.2182) -> (69.0644, 55.2182)
  line L337 (69.0644, 55.2182) -> (69.0644, 54.6932)
  line L338 (69.0644, 54.6932) -> (68.5019, 54.6932)
  line L339 (68.5019, 54.6932) -> (68.5019, 54.9557)
  line L340 (68.5019, 54.9557) -> (68.4644, 54.9557)
  line L341 (68.4644, 54.9557) -> (68.4644, 54.6932)
  line L342 (68.4644, 54.6932) -> (67.7894, 54.6932)
  line L343 (67.7894, 54.6932) -> (67.7894, 54.9557)
  line L344 (67.7894, 54.9557) -> (67.7519, 54.9557)
  line L345 (67.7519, 54.9557) -> (67.7519, 54.6932)
  line L346 (67.7519, 54.6932) -> (67.0957, 54.6932)
  line L347 (67.0957, 54.6932) -> (67.0957, 55.2182)
  line L348 (67.0957, 55.2182) -> (67.0581, 55.2182)
  line L349 (67.0581, 55.2182) -> (67.0581, 54.6932)
  line L350 (67.0581, 54.6932) -> (66.4394, 54.6932)
  line L351 (66.4394, 54.6932) -> (66.4394, 54.9557)
  line L352 (66.4394, 54.9557) -> (66.4019, 54.9557)
  line L353 (66.4019, 54.9557) -> (66.4019, 54.6932)
  line L354 (66.4019, 54.6932) -> (65.7644, 54.6932)
  line L355 (65.7644, 54.6932) -> (65.7644, 54.9557)
  line L356 (65.7644, 54.9557) -> (65.7269, 54.9557)
  line L357 (65.7269, 54.9557) -> (65.7269, 54.6932)
  line L358 (65.7269, 54.6932) -> (65.0894, 54.6932)
  line L359 (65.0894, 54.6932) -> (65.0894, 55.2182)
  line L360 (65.0894, 55.2182) -> (65.0519, 55.2182)
  line L361 (65.0519, 55.2182) -> (65.0519, 54.6932)
  line L362 (65.0519, 54.6932) -> (65.031, 54.6949)
  line L363 (65.031, 54.6949) -> (64.97, 54.716)
  line L364 (64.97, 54.716) -> (64.9046, 54.7653)
  line L365 (64.9046, 54.7653) -> (64.8611, 54.835)
  line L366 (64.8611, 54.835) -> (64.8453, 54.8975)
  line L367 (64.8453, 54.8975) -> (64.8454, 54.9182)
  line L368 (64.8454, 54.9182) -> (64.8454, 55.2402)
  line L369 (64.8454, 55.2402) -> (64.863, 55.3059)
  line L370 (64.863, 55.3059) -> (64.9113, 55.3774)
  line L371 (64.9113, 55.3774) -> (64.9827, 55.4256)
  line L372 (64.9827, 55.4256) -> (65.0483, 55.4432)
  line L373 (66.9366, 56.7178) -> (66.9548, 56.602)
  line L374 (66.9548, 56.602) -> (67.045, 56.6668)
  line L375 (67.045, 56.6668) -> (67.0916, 56.5604)
  line L376 (67.0916, 56.5604) -> (67.1624, 56.6492)
  line L377 (67.1624, 56.6492) -> (67.2338, 56.5604)
  line L378 (67.2338, 56.5604) -> (67.2798, 56.6668)
  line L379 (67.2798, 56.6668) -> (67.3707, 56.602)
  line L380 (67.3707, 56.602) -> (67.3886, 56.7178)
  line L381 (67.3886, 56.7178) -> (67.4918, 56.6803)
  line L382 (67.4918, 56.6803) -> (67.4804, 56.7973)
  line L383 (67.4804, 56.7973) -> (67.5888, 56.7932)
  line L384 (67.5888, 56.7932) -> (67.5488, 56.9024)
  line L385 (67.5488, 56.9024) -> (67.6541, 56.9301)
  line L386 (67.6541, 56.9301) -> (67.5884, 57.0235)
  line L387 (67.5884, 57.0235) -> (67.683, 57.0809)
  line L388 (67.683, 57.0809) -> (67.5964, 57.1518)
  line L389 (67.5964, 57.1518) -> (67.6736, 57.2346)
  line L390 (67.6736, 57.2346) -> (67.5724, 57.2774)
  line L391 (67.5724, 57.2774) -> (67.6259, 57.3797)
  line L392 (67.6259, 57.3797) -> (67.5179, 57.3912)
  line L393 (67.5179, 57.3912) -> (67.5439, 57.5057)
  line L394 (67.5439, 57.5057) -> (67.437, 57.4854)
  line L395 (67.437, 57.4854) -> (67.4336, 57.6031)
  line L396 (67.4336, 57.6031) -> (67.3357, 57.5522)
  line L397 (67.3357, 57.5522) -> (67.3035, 57.6647)
  line L398 (67.3035, 57.6647) -> (67.2218, 57.5872)
  line L399 (67.2218, 57.5872) -> (67.1624, 57.6858)
  line L400 (67.1624, 57.6858) -> (67.1033, 57.5872)
  line L401 (67.1033, 57.5872) -> (67.0218, 57.6647)
  line L402 (67.0218, 57.6647) -> (66.9892, 57.5522)
  line L403 (66.9892, 57.5522) -> (66.8914, 57.6031)
  line L404 (66.8914, 57.6031) -> (66.888, 57.4854)
  line L405 (66.888, 57.4854) -> (66.7812, 57.5057)
  line L406 (66.7812, 57.5057) -> (66.8074, 57.3912)
  line L407 (66.8074, 57.3912) -> (66.6989, 57.3797)
  line L408 (66.6989, 57.3797) -> (66.7527, 57.2774)
  line L409 (66.7527, 57.2774) -> (66.6517, 57.2346)
  line L410 (66.6517, 57.2346) -> (66.7286, 57.1518)
  line L411 (66.7286, 57.1518) -> (66.642, 57.0809)
  line L412 (66.642, 57.0809) -> (66.7368, 57.0235)
  line L413 (66.7368, 57.0235) -> (66.6709, 56.9301)
  line L414 (66.6709, 56.9301) -> (66.7763, 56.9024)
  line L415 (66.7763, 56.9024) -> (66.7361, 56.7932)
  line L416 (66.7361, 56.7932) -> (66.8448, 56.7973)
  line L417 (66.8448, 56.7973) -> (66.8331, 56.6803)
  line L418 (66.8331, 56.6803) -> (66.9366, 56.7178)
  line L419 (67.8974, 57.2961) -> (67.9025, 57.1147)
  line L420 (67.9025, 57.1147) -> (67.8716, 56.9356)
  line L421 (67.8716, 56.9356) -> (67.8603, 56.9008)
  line L422 (67.8603, 56.9008) -> (67.8536, 56.8786)
  line L423 (67.8536, 56.8786) -> (67.8052, 56.7606)
  line L424 (67.8052, 56.7606) -> (67.7283, 56.6047)
  line L425 (67.7283, 56.6047) -> (67.7074, 56.5633)
  line L426 (67.7074, 56.5633) -> (67.6961, 56.5412)
  line L427 (67.6961, 56.5412) -> (67.6609, 56.4753)
  line L428 (67.6609, 56.4753) -> (67.6295, 56.418)
  line L429 (67.6295, 56.418) -> (67.6062, 56.3717)
  line L430 (67.6062, 56.3717) -> (67.5896, 56.3309)
  line L431 (67.5896, 56.3309) -> (67.5847, 56.317)
  line L432 (67.5847, 56.317) -> (67.5757, 56.2924)
  line L433 (67.5757, 56.2924) -> (67.5243, 56.0358)
  line L434 (67.5243, 56.0358) -> (67.5232, 56.0094)
  line L435 (67.5232, 56.0094) -> (67.5232, 55.9169)
  line L436 (67.5232, 55.9169) -> (67.5191, 55.7057)
  line L437 (67.5191, 55.7057) -> (66.7241, 55.7057)
  line L438 (66.7241, 55.7057) -> (66.7263, 55.9783)
  line L439 (66.7263, 55.9783) -> (66.725, 56.0123)
  line L440 (66.725, 56.0123) -> (66.674, 56.3462)
  line L441 (66.674, 56.3462) -> (66.6651, 56.3787)
  line L442 (66.6651, 56.3787) -> (66.6648, 56.3795)
  line L443 (66.6648, 56.3795) -> (66.6615, 56.3881)
  line L444 (66.6615, 56.3881) -> (66.6615, 56.3912)
  line L445 (66.6615, 56.3912) -> (66.6554, 56.4119)
  line L446 (66.6554, 56.4119) -> (66.5615, 56.6041)
  line L447 (66.5615, 56.6041) -> (66.549, 56.6215)
  line L448 (66.549, 56.6215) -> (66.5304, 56.6492)
  line L449 (66.5304, 56.6492) -> (66.4546, 56.7963)
  line L450 (66.4546, 56.7963) -> (66.4023, 56.9532)
  line L451 (66.4023, 56.9532) -> (66.3956, 56.9856)
  line L452 (66.3956, 56.9856) -> (66.391, 57.0104)
  line L453 (66.391, 57.0104) -> (66.391, 57.2608)
  line L454 (66.391, 57.2608) -> (66.3956, 57.2856)
  line L455 (66.3956, 57.2856) -> (66.3996, 57.3059)
  line L456 (66.3996, 57.3059) -> (66.4711, 57.4987)
  line L457 (66.4711, 57.4987) -> (66.4812, 57.5166)
  line L458 (66.4812, 57.5166) -> (66.4929, 57.5375)
  line L459 (66.4929, 57.5375) -> (66.6464, 57.7174)
  line L460 (66.6464, 57.7174) -> (66.6651, 57.7322)
  line L461 (66.6651, 57.7322) -> (66.7003, 57.7633)
  line L462 (66.7003, 57.7633) -> (66.822, 57.8385)
  line L463 (66.822, 57.8385) -> (66.9978, 57.9008)
  line L464 (66.9978, 57.9008) -> (67.1834, 57.9174)
  line L465 (67.1834, 57.9174) -> (67.3252, 57.8996)
  line L466 (67.3252, 57.8996) -> (67.3703, 57.886)
  line L467 (67.3703, 57.886) -> (67.4194, 57.876)
  line L468 (67.4194, 57.876) -> (67.5615, 57.8151)
  line L469 (67.5615, 57.8151) -> (67.7187, 57.6921)
  line L470 (67.7187, 57.6921) -> (67.8318, 57.5276)
  line L471 (67.8318, 57.5276) -> (67.8841, 57.3821)
  line L472 (67.8841, 57.3821) -> (67.8912, 57.3321)
  line L473 (67.8912, 57.3321) -> (67.8974, 57.2961)
  line L474 (59.8394, 50.2176) -> (59.5556, 51.2717)
  line L475 (59.5556, 51.2717) -> (59.5556, 50.2176)
  line L476 (59.5556, 50.2176) -> (59.2181, 50.2176)
  line L477 (59.2181, 50.2176) -> (59.2181, 51.6932)
  line L478 (59.2181, 51.6932) -> (59.8095, 51.6932)
  line L479 (59.8095, 51.6932) -> (60.0236, 50.9098)
  line L480 (60.0236, 50.9098) -> (60.2277, 51.6932)
  line L481 (60.2277, 51.6932) -> (60.8212, 51.6932)
  line L482 (60.8212, 51.6932) -> (60.8212, 50.2188)
  line L483 (60.8212, 50.2188) -> (60.4019, 50.2188)
  line L484 (60.4019, 50.2188) -> (60.4019, 51.2717)
  line L485 (60.4019, 51.2717) -> (60.1294, 50.2176)
  line L486 (60.1294, 50.2176) -> (59.8394, 50.2176)
  line L487 (61.8859, 50.8307) -> (61.7665, 51.2586)
  line L488 (61.7665, 51.2586) -> (61.647, 50.8307)
  line L489 (61.647, 50.8307) -> (61.8859, 50.8307)
  line L490 (61.4816, 50.2176) -> (61.1144, 50.2176)
  line L491 (61.1144, 50.2176) -> (61.5693, 51.6932)
  line L492 (61.5693, 51.6932) -> (62.0478, 51.6932)
  line L493 (62.0478, 51.6932) -> (62.5107, 50.2188)
  line L494 (62.5107, 50.2188) -> (62.0486, 50.2176)
  line L495 (62.0486, 50.2176) -> (61.9654, 50.5083)
  line L496 (61.9654, 50.5083) -> (61.5701, 50.5083)
  line L497 (61.5701, 50.5083) -> (61.4816, 50.2176)
  line L498 (62.8019, 51.6932) -> (63.2286, 51.6932)
  line L499 (63.2286, 51.6932) -> (63.2286, 51.0834)
  line L500 (63.2286, 51.0834) -> (63.6367, 51.6932)
  line L501 (63.6367, 51.6932) -> (64.0437, 51.6932)
  line L502 (64.0437, 51.6932) -> (63.6712, 51.1536)
  line L503 (63.6712, 51.1536) -> (64.1331, 50.2176)
  line L504 (64.1331, 50.2176) -> (63.6378, 50.2176)
  line L505 (63.6378, 50.2176) -> (63.3832, 50.7748)
  line L506 (63.3832, 50.7748) -> (63.2302, 50.5576)
  line L507 (63.2302, 50.5576) -> (63.2302, 50.2176)
  line L508 (63.2302, 50.2176) -> (62.8019, 50.2176)
  line L509 (62.8019, 50.2176) -> (62.8019, 51.6932)
  line L510 (64.8554, 50.8116) -> (64.8554, 50.5682)
  line L511 (64.8554, 50.5682) -> (65.5207, 50.5682)
  line L512 (65.5207, 50.5682) -> (65.5207, 50.216)
  line L513 (65.5207, 50.216) -> (64.4115, 50.216)
  line L514 (64.4115, 50.216) -> (64.4115, 51.6932)
  line L515 (64.4115, 51.6932) -> (65.5207, 51.6932)
  line L516 (65.5207, 51.6932) -> (65.5207, 51.3531)
  line L517 (65.5207, 51.3531) -> (64.8554, 51.3531)
  line L518 (64.8554, 51.3531) -> (64.8554, 51.1389)
  line L519 (64.8554, 51.1389) -> (65.3933, 51.1389)
  line L520 (65.3933, 51.1389) -> (65.3933, 50.8116)
  line L521 (65.3933, 50.8116) -> (64.8554, 50.8116)
  line L522 (66.6302, 51.1262) -> (66.6405, 51.1326)
  line L523 (66.6405, 51.1326) -> (66.6492, 51.1385)
  line L524 (66.6492, 51.1385) -> (66.68, 51.1781)
  line L525 (66.68, 51.1781) -> (66.6927, 51.2268)
  line L526 (66.6927, 51.2268) -> (66.6923, 51.2371)
  line L527 (66.6923, 51.2371) -> (66.6923, 51.2639)
  line L528 (66.6923, 51.2639) -> (66.6488, 51.3436)
  line L529 (66.6488, 51.3436) -> (66.5511, 51.379)
  line L530 (66.5511, 51.379) -> (66.3101, 51.379)
  line L531 (66.3101, 51.379) -> (66.3101, 51.0969)
  line L532 (66.3101, 51.0969) -> (66.5032, 51.0969)
  line L533 (66.5032, 51.0969) -> (66.5152, 51.0964)
  line L534 (66.5152, 51.0964) -> (66.6302, 51.1262)
  line L535 (66.999, 51.5938) -> (67.0226, 51.5739)
  line L536 (67.0226, 51.5739) -> (67.0458, 51.5546)
  line L537 (67.0458, 51.5546) -> (67.1296, 51.4328)
  line L538 (67.1296, 51.4328) -> (67.1646, 51.2893)
  line L539 (67.1646, 51.2893) -> (67.1636, 51.259)
  line L540 (67.1636, 51.259) -> (67.164, 51.2395)
  line L541 (67.164, 51.2395) -> (67.1206, 51.0514)
  line L542 (67.1206, 51.0514) -> (67.1119, 51.034)
  line L543 (67.1119, 51.034) -> (67.103, 51.0178)
  line L544 (67.103, 51.0178) -> (67.0336, 50.9422)
  line L545 (67.0336, 50.9422) -> (66.9284, 50.8742)
  line L546 (66.9284, 50.8742) -> (66.9023, 50.8617)
  line L547 (66.9023, 50.8617) -> (67.1701, 50.2176)
  line L548 (67.1701, 50.2176) -> (66.6683, 50.2176)
  line L549 (66.6683, 50.2176) -> (66.4527, 50.7801)
  line L550 (66.4527, 50.7801) -> (66.3101, 50.7801)
  line L551 (66.3101, 50.7801) -> (66.3101, 50.2176)
  line L552 (66.3101, 50.2176) -> (65.8575, 50.2176)
  line L553 (65.8575, 50.2176) -> (65.8575, 51.6932)
  line L554 (65.8575, 51.6932) -> (66.6834, 51.6932)
  line L555 (66.6834, 51.6932) -> (66.8531, 51.6635)
  line L556 (66.8531, 51.6635) -> (66.999, 51.5938)
  line L557 (68.7919, 51.6932) -> (68.7919, 50.2188)
  line L558 (68.7919, 50.2188) -> (68.3392, 50.2188)
  line L559 (68.3392, 50.2188) -> (68.3392, 50.7909)
  line L560 (68.3392, 50.7909) -> (67.9935, 50.7909)
  line L561 (67.9935, 50.7909) -> (67.9935, 50.2176)
  line L562 (67.9935, 50.2176) -> (67.5408, 50.2176)
  line L563 (67.5408, 50.2176) -> (67.5408, 51.6932)
  line L564 (67.5408, 51.6932) -> (67.9935, 51.6932)
  line L565 (67.9935, 51.6932) -> (67.9935, 51.151)
  line L566 (67.9935, 51.151) -> (68.3392, 51.151)
  line L567 (68.3392, 51.151) -> (68.3392, 51.6932)
  line L568 (68.3392, 51.6932) -> (68.7919, 51.6932)
  line L569 (69.8554, 50.8307) -> (69.736, 51.2586)
  line L570 (69.736, 51.2586) -> (69.617, 50.8307)
  line L571 (69.617, 50.8307) -> (69.8554, 50.8307)
  line L572 (69.5396, 50.5083) -> (69.4511, 50.2176)
  line L573 (69.4511, 50.2176) -> (69.0835, 50.2176)
  line L574 (69.0835, 50.2176) -> (69.5388, 51.6932)
  line L575 (69.5388, 51.6932) -> (70.0177, 51.6932)
  line L576 (70.0177, 51.6932) -> (70.48, 50.2188)
  line L577 (70.48, 50.2188) -> (70.0181, 50.2176)
  line L578 (70.0181, 50.2176) -> (69.9349, 50.5083)
  line L579 (69.9349, 50.5083) -> (69.5396, 50.5083)
  line L580 (71.8394, 51.6932) -> (71.8394, 51.3422)
  line L581 (71.8394, 51.3422) -> (71.2136, 51.3422)
  line L582 (71.2136, 51.3422) -> (71.2136, 51.1022)
  line L583 (71.2136, 51.1022) -> (71.6943, 51.1022)
  line L584 (71.6943, 51.1022) -> (71.6943, 50.7695)
  line L585 (71.6943, 50.7695) -> (71.2136, 50.7695)
  line L586 (71.2136, 50.7695) -> (71.2136, 50.2176)
  line L587 (71.2136, 50.2176) -> (70.773, 50.2176)
  line L588 (70.773, 50.2176) -> (70.773, 51.6932)
  line L589 (70.773, 51.6932) -> (71.8394, 51.6932)
  line L590 (72.5843, 51.1389) -> (73.122, 51.1389)
  line L591 (73.122, 51.1389) -> (73.122, 50.8116)
  line L592 (73.122, 50.8116) -> (72.5843, 50.8116)
  line L593 (72.5843, 50.8116) -> (72.5843, 50.5682)
  line L594 (72.5843, 50.5682) -> (73.2495, 50.5682)
  line L595 (73.2495, 50.5682) -> (73.2495, 50.216)
  line L596 (73.2495, 50.216) -> (72.1394, 50.216)
  line L597 (72.1394, 50.216) -> (72.1394, 51.6932)
  line L598 (72.1394, 51.6932) -> (73.2495, 51.6932)
  line L599 (73.2495, 51.6932) -> (73.2495, 51.3531)
  line L600 (73.2495, 51.3531) -> (72.5843, 51.3531)
  line L601 (72.5843, 51.3531) -> (72.5843, 51.1389)
  line L602 (73.9232, 51.1529) -> (73.9545, 50.9514)
  line L603 (73.9545, 50.9514) -> (73.9552, 50.9309)
  line L604 (73.9552, 50.9309) -> (73.9552, 50.2184)
  line L605 (73.9552, 50.2184) -> (73.5876, 50.2184)
  line L606 (73.5876, 50.2184) -> (73.5876, 51.6932)
  line L607 (73.5876, 51.6932) -> (74.0144, 51.6932)
  line L608 (74.0144, 51.6932) -> (74.3579, 51.1532)
  line L609 (74.3579, 51.1532) -> (74.3726, 51.1307)
  line L610 (74.3726, 51.1307) -> (74.5025, 50.8948)
  line L611 (74.5025, 50.8948) -> (74.5136, 50.8702)
  line L612 (74.5136, 50.8702) -> (74.5078, 50.9022)
  line L613 (74.5078, 50.9022) -> (74.479, 51.1682)
  line L614 (74.479, 51.1682) -> (74.479, 51.6932)
  line L615 (74.479, 51.6932) -> (74.8474, 51.6932)
  line L616 (74.8474, 51.6932) -> (74.8466, 50.2176)
  line L617 (74.8466, 50.2176) -> (74.4783, 50.2176)
  line L618 (74.4783, 50.2176) -> (74.0745, 50.8682)
  line L619 (74.0745, 50.8682) -> (74.0597, 50.8928)
  line L620 (74.0597, 50.8928) -> (73.929, 51.1465)
  line L621 (73.929, 51.1465) -> (73.9177, 51.1727)
  line L622 (73.9177, 51.1727) -> (73.9232, 51.1529)
extrude "Extrude1" add sketch "Boden" along normal blind 5 makes body 1 in component "Boden"
fillet "Fillet1" radius 2 25 edges at (150, 2.5, -10) (137, 2.5, -10) (150, 2.5, -20) (127, 2.5, -10) (114, 2.5, -10) (114, 2.5, -20) (127, 2.5, -15) (137, 2.5, -15) (137, 2.5, -29) (127, 2.5, -29) (155, 2.5, -29) (109, 2.5, -29) (149, 2.5, -65) (135, 2.5, -65) (129, 2.5, -65) (115, 2.5, -65) (115, 2.5, -85) (129, 2.5, -75) (135, 2.5, -75) (149, 2.5, -85) (132, 2.5, -84.0491) (147, 2.5, -94) (117, 2.5, -94) (147, 2.5, -104) (117, 2.5, -104) on bodies 1 in component "Boden"
extrude "Extrude1'" add sketch "Halter" along normal blind 5 separate body makes body 2 in component "Halter"
extrude "Extrude1''" add sketch "Seiten" along normal blind 5 separate body makes body 3 in component "Seite"
fillet "Fillet1'" radius 2.5 9 edges at (12, 2.5, -62) (15.5, 2.5, -66) (26, 2.5, -48) (34, 2.5, -66) (23, 2.5, -43) (12, 2.5, -20) (12, 2.5, -81) (12, 2.5, -100) (32.5, 2.5, -81) on bodies 3 in component "Seite"
extrude "Extrude1'''" add sketch "Hebel" along normal blind 5 separate body makes body 4 in component "Hebel"
extrude "Extrude2" cut sketch "Sketch8" along normal blind 1 bodies 4 in component "Hebel"
fillet "Fillet1''" radius 2 8 edges at (62, 2.5, -81) (72, 2.5, -81) (56.5, 2.5, -90) (77.5, 2.5, -90) (62, 2.5, -105.0296) (72, 2.5, -105.0296) (72, 2.5, -100) (62, 2.5, -100) on bodies 4 in component "Hebel"
extrude "Extrude1''''" add sketch "Quer" along normal blind 5 separate body makes body 5 in component "Quer"